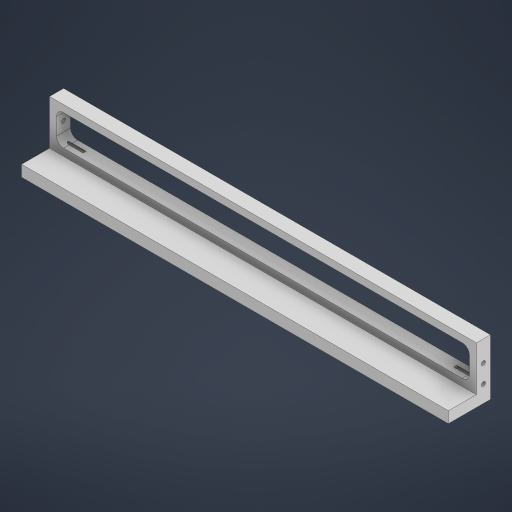
# Autodesk Inventor part: chessboard-base-2
Saved by Autodesk Inventor 2023 (Build 270158000, 158)
## iProperties
Created: 2023-12-20
Part Number: chessboard-base-2
Material: Generic
Document SubType Name: Modeling
Designer: hrush
Density: 1 g/cm^3
Appearance: Default
Author: hrush
Autodesk Inventor part; units mm, degrees
ref_plane "YZ Plane" through (0, 0, 0) normal (1, 0, 0) x (0, 1, 0)
ref_plane "XZ Plane" through (0, 0, 0) normal (0, 1, 0) x (-1, 0, 0)
ref_plane "XY Plane" through (0, 0, 0) normal (0, 0, 1) x (1, 0, 0)
sketch "Sketch1" plane through (0, 0, 0) normal (0, 1, 0) x (-1, 0, 0)
  line L0 (0, 0) -> (305, 0)
  line L1 (305, 0) -> (305, -10)
  line L2 (305, -10) -> (0, -10)
  line L3 (0, -10) -> (0, 0)
  dimension "d0" = 305
  dimension "d1" = 10
  constraints: 8 end point, 2 parallel, 1 horizontal, 1 perpendicular
  measures "d0" distance of L1.end L2.end
  measures "d1" distance of L0.end L1.end
extrude "Extrusion1" add sketch "Sketch1" along normal blind 40
sketch "Sketch2" plane through (-305, 0, 0) normal (0, 0, 1) x (1, 0, 0)
  line L0 (305, 0) -> (0, 0) projected
  line L1 (305, 0) -> (305, 40) projected
  line L2 (0, 0) -> (305, 0)
  line L3 (305, 0) -> (305, 8)
  line L4 (305, 8) -> (0, 8)
  line L5 (0, 8) -> (0, 0)
  dimension "d4" = 8
  constraints: 8 end point, 2 parallel, 1 horizontal, 1 perpendicular, 1 point on line
  measures "d4" distance of L3.end L2.end
extrude "Extrusion2" add sketch "Sketch2" along normal blind 20
sketch "Sketch3" plane through (-305, 40, 0) normal (0, 0, 1) x (1, 0, 0)
  line L0 (305, -27) -> (0, -27) projected
  line L1 (5, -5) -> (300, -5)
  line L2 (300, -5) -> (300, -27)
  line L3 (300, -27) -> (5, -27)
  line L4 (5, -27) -> (5, -5)
  line L5 (0, -32) -> (0, 0) projected
  line L6 (0, 0) -> (305, 0) projected
  line L7 (305, -32) -> (305, 0) projected
  point P0 (305, -40)
  point P1 (305, -16)
  dimension "d8" = 5
  dimension "d9" = 5
  dimension "d10" = 5
  constraints: 8 end point, 2 parallel, 1 horizontal, 1 midpoint, 1 perpendicular, 1 point on line
  measures "d8" distance between parallel lines of L5 L4
  measures "d9" distance between parallel lines of L6 L1
  measures "d10" distance from line of point (305, -16) L2
extrude "Extrusion3" cut sketch "Sketch3" against normal blind 20 contours L0 L4 L1 L2
fillet "Fillet2" radius 5 4 edges at (-300, 13, -5) (-300, 35, -5) (-5, 13, -5) (-5, 35, -5)
sketch "Sketch4" plane through (-305, 0, -10) normal (-1, 0, 0) x (0, 0, 1)
  circle A0 centre (5, 25) radius 1.5
  circle A1 centre (5, 12) radius 1.5
  line L0 (0, 40) -> (10, 40) projected
  line L1 (0, 0) -> (0, 40) projected
  point P0 (10, 0)
  dimension "d14" = 3
  dimension "d15" = 3
  dimension "d16" = 15
  dimension "d17" = 10
  dimension "d18" = 5
  dimension "d19" = 5
  constraints: 2 centre point
  measures "d14" diameter of A0
  measures "d15" diameter of A1
  measures "d16" distance from line of L0 A0.centre
  measures "d18" distance from line of L1 A1.centre
  measures "d19" distance from line of L1 A0.centre
extrude "Extrusion4" cut sketch "Sketch4" against normal blind 20
sketch "Sketch5" plane through (0, 0, -10) normal (1, 0, 0) x (0, 0, -1)
  circle A0 centre (-5, 25) radius 1.5
  circle A1 centre (-5, 12) radius 1.5
  line L0 (0, 0) -> (0, 40) projected
  line L1 (-10, 40) -> (0, 40) projected
  point P0 (-10, 0)
  dimension "d22" = 3
  dimension "d23" = 3
  dimension "d24" = 5
  dimension "d25" = 5
  dimension "d26" = 10
  dimension "d27" = 15
  constraints: 2 centre point
  measures "d22" diameter of A0
  measures "d23" diameter of A1
  measures "d24" distance from line of L0 A0.centre
  measures "d25" distance from line of L0 A1.centre
  measures "d27" distance from line of A0.centre L1
extrude "Extrusion5" cut sketch "Sketch5" against normal blind 20
thread "Thread1" size "M3x0.5" class "6H" standard "ANSI Metric M Profile" full length
thread "Thread2" size "M3x0.5" class "6H" standard "ANSI Metric M Profile" full length
thread "Thread3" size "M3x0.5" class "6H" standard "ANSI Metric M Profile" full length
thread "Thread4" size "M3x0.5" class "6H" standard "ANSI Metric M Profile" full length
body "Solid1"
